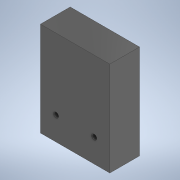
# Autodesk Inventor part: backmotormount
Saved by Autodesk Inventor 2021.5 (Build 255421000, 421)
## iProperties
Created: 2024-11-18
Part Number: backmotormount
Material: Wood (Birch)
Document SubType Name: Modeling
Designer: email
Density: 0.55 g/cm^3
Appearance: Birch - Natural Polished
Author: email
Autodesk Inventor part; units mm, degrees
ref_plane "YZ Plane" through (0, 0, 0) normal (1, 0, 0) x (0, 1, 0)
ref_plane "XZ Plane" through (0, 0, 0) normal (0, 1, 0) x (-1, 0, 0)
ref_plane "XY Plane" through (0, 0, 0) normal (0, 0, 1) x (1, 0, 0)
sketch "Sketch1" plane through (0, 0, 0) normal (0, 1, 0) x (-1, 0, 0)
  line L0 (0, 0) -> (-88.9, 0)
  line L1 (-88.9, 0) -> (-88.9, -38.1)
  line L2 (-88.9, -38.1) -> (0, -38.1)
  line L3 (0, -38.1) -> (0, 0)
  dimension "d0" = 88.9
  dimension "d1" = 38.1
  constraints: 8 end point, 2 parallel, 1 horizontal, 1 perpendicular
  measures "d0" distance between parallel lines of L1 L3
  measures "d1" distance of L0.end L1.end
extrude "Extrusion1" add sketch "Sketch1" along normal blind 120.9926
sketch "Sketch2" plane through (0, 0, 0) normal (0, 0, 1) x (1, 0, 0)
  line L0 (88.9, 0) -> (0, 0) construction
  line L1 (0, 0) -> (20, 0) construction
  line L2 (20, 0) -> (20, 30) construction
  line L3 (20, 30) -> (0, 30) construction
  line L4 (0, 30) -> (0, 0) construction
  line L5 (88.9, 0) -> (68.9, 0) construction
  line L6 (68.9, 0) -> (68.9, 30) construction
  line L7 (68.9, 30) -> (88.9, 30) construction
  line L8 (88.9, 30) -> (88.9, 0) construction
  circle A0 centre (20, 30) radius 3
  circle A1 centre (68.9, 30) radius 3
  dimension "d4" = 20
  dimension "d5" = 20
  dimension "d6" = 30
  dimension "d7" = 30
  dimension "d8" = 6
  dimension "d9" = 6
  dimension "d17" = 48.9
  constraints: 16 end point, 4 parallel, 2 centre point, 2 coincident, 2 horizontal, 2 perpendicular, 1 point on line
  measures "d4" distance of L6.end L7.end
  measures "d5" distance of L2.end L3.end
  measures "d6" distance of L1.end L2.end
  measures "d7" distance of L5.end L6.end
  measures "d8" diameter of A0
  measures "d9" diameter of A1
  measures "d17" distance of L2.end L6.end
hole "Hole1" at (68.9, 30, 0) at (20, 30, 0) direction (0, 0, -1) diameter 6.5 end through all
body "Solid1"
